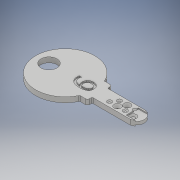
# Autodesk Inventor part: TSA006_stubby
Saved by Autodesk Inventor 2018 (Build 220112000, 112)
## iProperties
Created: 2018-08-22
Part Number: TSA006_stubby
Material: Generic
Document SubType Name: Modeling
Designer: Fatts
Density: 1 g/cm^3
Appearance: Default
Author: Fatts
Autodesk Inventor part; units mm, degrees
ref_plane "YZ Plane" through (0, 0, 0) normal (1, 0, 0) x (0, 1, 0)
ref_plane "XZ Plane" through (0, 0, 0) normal (0, 1, 0) x (-1, 0, 0)
ref_plane "XY Plane" through (0, 0, 0) normal (0, 0, 1) x (1, 0, 0)
sketch "Sketch1" plane through (0, 0, 0) normal (0, 1, 0) x (-1, 0, 0)
  line L0 (3.048, 7.366) -> (3.048, -7.366)
  line L1 (-3.048, 7.366) -> (-3.048, -7.366)
  line L2 (3.048, 0) -> (-3.048, 0) construction
  line L3 (3.048, -7.366) -> (-3.048, -7.366) construction
  arc A0 (-3.048, -7.366) -> (3.048, -7.366) centre (0, -6.7917) ccw
  line L4 (4.9022, 8.636) -> (4.9022, 10.6426)
  line L5 (-4.9022, 10.6426) -> (-4.9022, 8.636)
  line L6 (4.9022, 9.6393) -> (-4.9022, 9.6393) construction
  line L7 (0, 0) -> (0, 9.6393) construction
  line L8 (-4.0132, 7.747) -> (-3.429, 7.747)
  line L9 (3.429, 7.747) -> (4.0132, 7.747)
  arc A1 (4.0132, 7.747) -> (4.9022, 8.636) centre (4.0132, 8.636) ccw
  arc A2 (-4.9022, 8.636) -> (-4.0132, 7.747) centre (-4.0132, 8.636) ccw
  arc A3 (3.429, 7.747) -> (3.048, 7.366) centre (3.429, 7.366) ccw
  arc A4 (-3.048, 7.366) -> (-3.429, 7.747) centre (-3.429, 7.366) ccw
  line L10 (-11.7228, 21.4884) -> (11.7228, 21.4884) construction
  line L11 (0, 9.6393) -> (0, 21.4884) construction
  arc A5 (-4.9022, 10.6426) -> (-5.2832, 11.0236) centre (-5.2832, 10.6426) ccw
  arc A6 (5.2832, 11.0236) -> (4.9022, 10.6426) centre (5.2832, 10.6426) ccw
  line L12 (0, 21.4884) -> (0, 33.2112) construction
  line L13 (-5.2832, 11.0236) -> (5.2832, 11.0236) construction
  arc A7 (5.2832, 11.0236) -> (-5.2832, 11.0236) centre (0, 21.4884) ccw
  point P0 (4.9022, 7.747)
  point P1 (4.9022, 11.0236)
  dimension "d1" = 6.096
  dimension "d2" = 2.5273
  dimension "d3" = 7.366
  dimension "d8" = 9.8044
  dimension "d9" = 3.2766
  dimension "d10" = 0.889
  dimension "d11" = 0.381
  dimension "d13" = 0.381
  dimension "d174" = 1.3843
  dimension "d175" = 9.6393
  dimension "d176" = 10.4648
  dimension "d189" = 20.9169
  constraints: 28 end point, 18 point on circle, 10 tangent, 8 centre point, 7 midpoint, 7 vertical, 6 horizontal, 3 equal radius, 3 point on line, 2 coincident, 1 collinear
  measures "d1" distance between parallel lines of L0 L1
  measures "d2" distance edge to line of A0 L3
  measures "d3" distance from line of point (0, 0) L3
  measures "d8" distance of L6.start L6.end
  measures "d9" distance of point (4.902, 7.747) point (4.902, 11.024)
  measures "d10" radius of A1
  measures "d11" radius of A3
  measures "d13" radius of A5
  measures "d174" distance between parallel lines of L6 L13
  measures "d175" distance from line of point (0, 0) L6
  measures "d176" distance from line of L13 A7.centre
extrude "MainBody" add sketch "Sketch1" along normal blind 2.02
sketch "Sketch7" plane through (0, 2.02, 0) normal (0, 1, 0) x (1, 0, 0)
  line L0 (-2.4536, 5.1435) -> (2.4536, 5.1435)
  line L1 (2.4536, 5.1435) -> (2.4536, 9.8933)
  line L2 (-2.4536, 5.1435) -> (-2.4536, 9.8933)
  line L3 (-2.4536, 9.8933) -> (2.4536, 9.8933)
  line L4 (0, 0) -> (0, 5.1435) construction
  dimension "d147" = 4.9073
  dimension "d148" = 9.8933
  dimension "d149" = 4.7498
  constraints: 10 end point, 2 perpendicular, 2 vertical, 1 horizontal, 1 midpoint
  measures "d147" distance of L0.start L0.end
  measures "d148" distance from line of L3 L4.start
  measures "d149" distance of L0.end L1.end
extrude "WardingTop" cut sketch "Sketch7" against normal blind 0.41
extrude "WardingBottom" cut sketch "Sketch7" along normal blind 0.41 from surface at -2.02
sketch "Sketch2" plane through (0, 2.02, 0) normal (0, 1, 0) x (1, 0, 0)
  circle A0 centre (0, -27.94) radius 3.175
  line L0 (0, 0) -> (0, -27.94) construction
  dimension "d177" = 6.35
  dimension "d178" = 27.94
  constraints: 2 end point, 1 centre point, 1 vertical
  measures "d177" diameter of A0
  measures "d178" distance of L0.start L0.end
extrude "RingHole" cut sketch "Sketch2" against normal through all
sketch "Sketch3" plane through (0, 2.02, 0) normal (0, 1, 0) x (1, 0, 0)
  line L0 (0, 0) -> (0, 9.8933) construction
  arc A0 (3.048, 7.366) -> (-3.048, 7.366) centre (0, 6.7917) ccw construction
  line L1 (-2.9336, 9.8933) -> (2.9336, 9.8933) construction
  circle A1 centre (1.1151, 3.4925) radius 0.889
  line L2 (3.048, -7.366) -> (3.048, 7.366) projected
  circle A2 centre (-1.1176, 5.1435) radius 0.889
  circle A3 centre (1.1151, -2.7559) radius 0.889
  circle A4 centre (-1.1176, -1.1049) radius 0.889
  point P0 (0, 9.8933)
  dimension "d21" = 1.9329
  dimension "d22" = 6.4008
  dimension "d23" = 1.778
  dimension "d24" = 1.778
  dimension "d25" = 4.7498
  dimension "d26" = 4.1656
  dimension "d27" = 1.778
  dimension "d28" = 1.9329
  dimension "d29" = 6.2484
  dimension "d30" = 1.778
  dimension "d31" = 4.1656
  dimension "d32" = 6.2484
  constraints: 4 centre point, 4 end point, 2 point on circle, 1 horizontal, 1 midpoint, 1 vertical
  measures "d21" distance from line of L2 A1.centre
  measures "d22" distance from line of L1 A1.centre
  measures "d23" diameter of A1
  measures "d24" diameter of A2
  measures "d25" distance from line of L1 A2.centre
  measures "d26" distance from line of L2 A2.centre
  measures "d27" diameter of A3
  measures "d28" distance from line of L2 A3.centre
  measures "d29" distance of A1.centre A3.centre
  measures "d30" diameter of A4
  measures "d31" distance from line of L2 A4.centre
  measures "d32" distance of A2.centre A4.centre
extrude "SmallDimpleTop" cut sketch "Sketch3" against normal blind 0.41
sketch "Sketch4" plane through (0, 2.02, 0) normal (0, 1, 0) x (1, 0, 0)
  line L0 (0, 0) -> (0, 9.8933) construction
  arc A0 (3.048, 7.366) -> (-3.048, 7.366) centre (0, 6.7917) ccw construction
  line L1 (-3.5523, 9.8933) -> (3.5523, 9.8933) construction
  circle A1 centre (1.1151, 0.3683) radius 1.3335
  line L2 (3.048, -7.366) -> (3.048, 7.366) construction
  circle A2 centre (-1.1176, 2.0193) radius 1.3335
  circle A3 centre (1.1176, 6.6167) radius 1.3335
  point P0 (0, 9.8933)
  dimension "d38" = 2.667
  dimension "d39" = 1.9329
  dimension "d40" = 9.525
  dimension "d41" = 2.667
  dimension "d42" = 4.1656
  dimension "d43" = 7.874
  dimension "d64" = 2.667
  dimension "d65" = 1.9304
  dimension "d66" = 6.2484
  constraints: 4 end point, 3 centre point, 2 point on circle, 1 horizontal, 1 midpoint, 1 vertical
  measures "d38" diameter of A1
  measures "d39" distance from line of L2 A1.centre
  measures "d40" distance from line of L1 A1.centre
  measures "d41" diameter of A2
  measures "d42" distance from line of L2 A2.centre
  measures "d43" distance from line of L1 A2.centre
  measures "d64" diameter of A3
  measures "d65" distance from line of A3.centre L2
  measures "d66" distance of A1.centre A3.centre
extrude "LargeDimpleTop" cut sketch "Sketch4" against normal blind 1.0033
sketch "Sketch5" plane through (0, 0, 0) normal (0, -1, 0) x (1, 0, 0)
  circle A0 centre (1.1151, 1.1049) radius 0.889
  circle A1 centre (-1.1176, 2.7559) radius 0.889
  circle A2 centre (1.1151, -5.1435) radius 0.889
  circle A3 centre (-1.1176, -3.4925) radius 0.889
  line L0 (0, 0) -> (0, -9.8933) construction
  arc A4 (-3.048, -7.366) -> (3.048, -7.366) centre (0, -6.7917) ccw construction
  line L1 (2.4831, -9.8933) -> (-2.4831, -9.8933) construction
  line L2 (-3.048, -7.366) -> (-3.048, 7.366) construction
  point P0 (0, -9.8933)
  dimension "d73" = 1.778
  dimension "d74" = 1.778
  dimension "d77" = 1.778
  dimension "d79" = 6.2484
  dimension "d80" = 1.778
  dimension "d82" = 6.2484
  dimension "d83" = 6.4008
  dimension "d84" = 4.7498
  dimension "d85" = 1.9304
  dimension "d86" = 4.1631
  dimension "d87" = 4.1631
  dimension "d88" = 1.9304
  constraints: 4 centre point, 4 end point, 2 point on circle, 1 horizontal, 1 midpoint, 1 vertical
  measures "d73" diameter of A0
  measures "d74" diameter of A1
  measures "d77" diameter of A2
  measures "d79" distance of A0.centre A2.centre
  measures "d80" diameter of A3
  measures "d82" distance of A1.centre A3.centre
  measures "d83" distance from line of L1 A3.centre
  measures "d84" distance from line of L1 A2.centre
  measures "d85" distance from line of L2 A3.centre
  measures "d86" distance from line of L2 A2.centre
  measures "d87" distance from line of L2 A0.centre
  measures "d88" distance from line of L2 A1.centre
extrude "SmallDimpleBottom" cut sketch "Sketch5" against normal blind 0.41
sketch "Sketch6" plane through (0, 0, 0) normal (0, -1, 0) x (1, 0, 0)
  circle A0 centre (-1.1176, -6.6167) radius 1.3335
  circle A1 centre (-1.1176, -0.3683) radius 1.3335
  circle A2 centre (1.1176, -2.0193) radius 1.3335
  line L0 (0, 0) -> (0, -9.8933) construction
  arc A3 (-3.048, -7.366) -> (3.048, -7.366) centre (0, -6.7917) ccw construction
  line L1 (3.7489, -9.8933) -> (-3.7489, -9.8933) construction
  line L2 (-3.048, -7.366) -> (-3.048, 7.366) construction
  point P0 (0, -9.8933)
  dimension "d91" = 2.667
  dimension "d92" = 2.667
  dimension "d93" = 2.667
  dimension "d95" = 1.9304
  dimension "d96" = 1.9304
  dimension "d97" = 6.2484
  dimension "d98" = 9.525
  dimension "d99" = 4.1656
  dimension "d100" = 7.874
  constraints: 4 end point, 3 centre point, 2 point on circle, 1 horizontal, 1 midpoint, 1 vertical
  measures "d91" diameter of A0
  measures "d92" diameter of A1
  measures "d93" diameter of A2
  measures "d95" distance from line of L2 A1.centre
  measures "d96" distance from line of L2 A0.centre
  measures "d97" distance of A0.centre A1.centre
  measures "d98" distance from line of L1 A1.centre
  measures "d99" distance from line of L2 A2.centre
  measures "d100" distance from line of L1 A2.centre
extrude "LargeDimpleBottom" cut sketch "Sketch6" against normal blind 1.0033
chamfer "SmallDimpleChamfer" distance 0.41 angle 45 8 edges at (1.1151, 0.41, -4.2545) (-2.0066, 0.41, -3.4925) (0.2261, 0.41, 1.1049) (-2.0066, 0.41, 2.7559) (-1.1176, 1.61, -4.2545) (0.2261, 1.61, -3.4925) (-2.0066, 1.61, 1.1049) (0.2261, 1.61, 2.7559)
chamfer "LargeDimpleChamfer" distance 1.0033 angle 45 4 edges at (-2.4511, 1.0167, -2.0193) (-0.2184, 1.0167, -0.3683) (-2.4511, 1.0033, -0.3683) (-0.2159, 1.0033, -2.0193)
chamfer "LargeWardingDimpleChamfer" distance 0.5933 angle 45 2 edges at (-2.4511, 1.0033, -6.6167) (-0.2159, 1.0167, -6.6167)
sketch "Sketch11" plane through (0, 2.02, 0) normal (0, 1, 0) x (1, 0, 0)
  line L0 (2.7352, -17.7393) -> (-2.7352, -17.7393) construction
  line L1 (-2.7352, -17.7393) -> (-2.7352, -10.16) construction
  line L2 (-2.7352, -10.16) -> (2.7352, -10.16) construction
  line L3 (2.7352, -10.16) -> (2.7352, -17.7393) construction
  line L4 (0, -10.16) -> (0, 0) construction
  spline S0 degree 2 poles (-2.4043, -12.6766) (-2.4043, -12.1154) (-2.0322, -11.1643) (-1.7191, -10.8453) knots 0 0 0 1 2 2 2
  spline S1 degree 2 poles (-1.7191, -10.8453) (-1.3942, -10.5085) (-0.5789, -10.16) (-0.0886, -10.16) knots 0 0 0 1 2 2 2
  spline S2 degree 2 poles (-0.0886, -10.16) (0.4017, -10.16) (1.211, -10.4908) (1.5182, -10.8216) knots 0 0 0 1 2 2 2
  spline S3 degree 2 poles (1.5182, -10.8216) (1.8963, -11.2174) (2.3216, -12.5466) (2.3216, -13.5154) knots 0 0 0 1 2 2 2
  spline S4 degree 2 poles (2.3216, -13.5154) (2.3216, -14.4665) (1.9317, -15.9966) (1.5241, -16.5637) knots 0 0 0 1 2 2 2
  spline S5 degree 2 poles (1.5241, -16.5637) (1.1283, -17.119) (-0.1241, -17.7393) (-0.9452, -17.7393) knots 0 0 0 1 2 2 2
  spline S6 degree 2 poles (-0.9452, -17.7393) (-1.1874, -17.7393) (-1.6127, -17.692) (-1.7722, -17.6388) knots 0 0 0 1 2 2 2
  line L5 (-1.7722, -17.6388) -> (-1.7722, -16.6996)
  line L6 (-1.7722, -16.6996) -> (-1.7309, -16.6996)
  spline S7 degree 2 poles (-1.7309, -16.6996) (-1.595, -16.7704) (-1.0988, -16.8945) (-0.8152, -16.8945) knots 0 0 0 1 2 2 2
  spline S8 degree 2 poles (-0.8152, -16.8945) (0.0945, -16.8945) (1.211, -15.6657) (1.3174, -14.4606) knots 0 0 0 1 2 2 2
  spline S9 degree 2 poles (1.3174, -14.4606) (0.9688, -14.7028) (0.2363, -14.9687) (-0.2009, -14.9687) knots 0 0 0 1 2 2 2
  spline S10 degree 2 poles (-0.2009, -14.9687) (-0.6262, -14.9687) (-1.2642, -14.7974) (-1.6127, -14.5374) knots 0 0 0 1 2 2 2
  spline S11 degree 2 poles (-1.6127, -14.5374) (-2.0144, -14.2361) (-2.4043, -13.3028) (-2.4043, -12.6766) knots 0 0 0 1 2 2 2
  spline S12 degree 2 poles (-1.4119, -12.6352) (-1.4119, -13.0842) (-1.1756, -13.6927) (-0.9157, -13.9053) knots 0 0 0 1 2 2 2
  spline S13 degree 2 poles (-0.9157, -13.9053) (-0.7207, -14.0589) (-0.2363, -14.1593) (0.0177, -14.1593) knots 0 0 0 1 2 2 2
  spline S14 degree 2 poles (0.0177, -14.1593) (0.3604, -14.1593) (1.0043, -13.9526) (1.3174, -13.7576) knots 0 0 0 1 2 2 2
  spline S15 degree 2 poles (1.3174, -13.7576) (1.3233, -13.6513) (1.3351, -13.4505) (1.3351, -13.2969) knots 0 0 0 1 2 2 2
  spline S16 degree 2 poles (1.3351, -13.2969) (1.3351, -12.5407) (1.0397, -11.6132) (0.8152, -11.371) knots 0 0 0 1 2 2 2
  spline S17 degree 2 poles (0.8152, -11.371) (0.6085, -11.1406) (0.1595, -10.9575) (-0.0945, -10.9575) knots 0 0 0 1 2 2 2
  spline S18 degree 2 poles (-0.0945, -10.9575) (-0.6853, -10.9575) (-1.4119, -11.7964) (-1.4119, -12.6352) knots 0 0 0 1 2 2 2
  dimension "d179" = 5.4703
  dimension "d180" = 7.5793
  dimension "d181" = 10.16
  constraints: 2 end point, 1 horizontal, 1 midpoint, 1 vertical, 2 other
  measures "d179" distance of L0.start L0.end
  measures "d180" distance of L0.end L1.end
  measures "d181" distance of L4.start L4.end
extrude "LogoTop" cut sketch "Sketch11" against normal blind 0.508
sketch "Sketch12" plane through (0, 0, 0) normal (0, -1, 0) x (1, 0, 0)
  line L0 (-2.7352, 17.7393) -> (2.7352, 17.7393) construction
  line L1 (2.7352, 17.7393) -> (2.7352, 10.16) construction
  line L2 (2.7352, 10.16) -> (-2.7352, 10.16) construction
  line L3 (-2.7352, 10.16) -> (-2.7352, 17.7393) construction
  line L4 (0, 10.16) -> (0, 0) construction
  spline S0 degree 2 poles (2.4043, 12.6766) (2.4043, 12.1154) (2.0322, 11.1643) (1.7191, 10.8453) knots 0 0 0 1 2 2 2
  spline S1 degree 2 poles (1.7191, 10.8453) (1.3942, 10.5085) (0.5789, 10.16) (0.0886, 10.16) knots 0 0 0 1 2 2 2
  spline S2 degree 2 poles (0.0886, 10.16) (-0.4017, 10.16) (-1.211, 10.4908) (-1.5182, 10.8216) knots 0 0 0 1 2 2 2
  spline S3 degree 2 poles (-1.5182, 10.8216) (-1.8963, 11.2174) (-2.3216, 12.5466) (-2.3216, 13.5154) knots 0 0 0 1 2 2 2
  spline S4 degree 2 poles (-2.3216, 13.5154) (-2.3216, 14.4665) (-1.9317, 15.9966) (-1.5241, 16.5637) knots 0 0 0 1 2 2 2
  spline S5 degree 2 poles (-1.5241, 16.5637) (-1.1283, 17.119) (0.1241, 17.7393) (0.9452, 17.7393) knots 0 0 0 1 2 2 2
  spline S6 degree 2 poles (0.9452, 17.7393) (1.1874, 17.7393) (1.6127, 17.692) (1.7722, 17.6388) knots 0 0 0 1 2 2 2
  line L5 (1.7722, 17.6388) -> (1.7722, 16.6996)
  line L6 (1.7722, 16.6996) -> (1.7309, 16.6996)
  spline S7 degree 2 poles (1.7309, 16.6996) (1.595, 16.7704) (1.0988, 16.8945) (0.8152, 16.8945) knots 0 0 0 1 2 2 2
  spline S8 degree 2 poles (0.8152, 16.8945) (-0.0945, 16.8945) (-1.211, 15.6657) (-1.3174, 14.4606) knots 0 0 0 1 2 2 2
  spline S9 degree 2 poles (-1.3174, 14.4606) (-0.9688, 14.7028) (-0.2363, 14.9687) (0.2009, 14.9687) knots 0 0 0 1 2 2 2
  spline S10 degree 2 poles (0.2009, 14.9687) (0.6262, 14.9687) (1.2642, 14.7974) (1.6127, 14.5374) knots 0 0 0 1 2 2 2
  spline S11 degree 2 poles (1.6127, 14.5374) (2.0144, 14.2361) (2.4043, 13.3028) (2.4043, 12.6766) knots 0 0 0 1 2 2 2
  spline S12 degree 2 poles (1.4119, 12.6352) (1.4119, 13.0842) (1.1756, 13.6927) (0.9157, 13.9053) knots 0 0 0 1 2 2 2
  spline S13 degree 2 poles (0.9157, 13.9053) (0.7207, 14.0589) (0.2363, 14.1593) (-0.0177, 14.1593) knots 0 0 0 1 2 2 2
  spline S14 degree 2 poles (-0.0177, 14.1593) (-0.3604, 14.1593) (-1.0043, 13.9526) (-1.3174, 13.7576) knots 0 0 0 1 2 2 2
  spline S15 degree 2 poles (-1.3174, 13.7576) (-1.3233, 13.6513) (-1.3351, 13.4505) (-1.3351, 13.2969) knots 0 0 0 1 2 2 2
  spline S16 degree 2 poles (-1.3351, 13.2969) (-1.3351, 12.5407) (-1.0397, 11.6132) (-0.8152, 11.371) knots 0 0 0 1 2 2 2
  spline S17 degree 2 poles (-0.8152, 11.371) (-0.6085, 11.1406) (-0.1595, 10.9575) (0.0945, 10.9575) knots 0 0 0 1 2 2 2
  spline S18 degree 2 poles (0.0945, 10.9575) (0.6853, 10.9575) (1.4119, 11.7964) (1.4119, 12.6352) knots 0 0 0 1 2 2 2
  dimension "d184" = 7.5793
  dimension "d185" = 5.4703
  dimension "d186" = 10.16
  constraints: 2 end point, 1 horizontal, 1 midpoint, 1 vertical, 2 other
  measures "d184" distance of L0.end L1.end
  measures "d185" distance of L0.start L0.end
  measures "d186" distance of L4.start L4.end
extrude "LogoBottom" cut sketch "Sketch12" against normal blind 0.508
body "Solid1"
